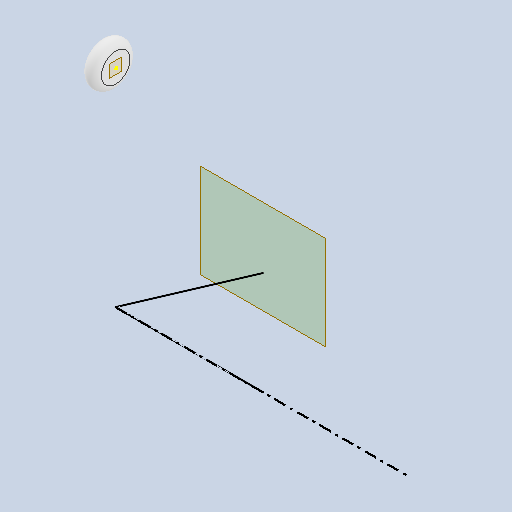
# Autodesk Inventor part: Landing Gear Wheel
Saved by Autodesk Inventor 2025 (Build 290162000, 162)
## iProperties
Created: 2024-09-17
Part Number: Landing Gear Wheel
Material: ABS Plastic
Document SubType Name: Modeling
Designer: Cupri
Density: 1.06 g/cm^3
Appearance: Smooth - White
Mass: 106.525 g
Surface Area: 124.48 cm^2
Volume: 100.495 cm^3
Author: Cupri
Autodesk Inventor part; units mm, degrees
ref_plane "YZ Plane" through (0, 0, 0) normal (1, 0, 0) x (0, 1, 0)
ref_plane "XZ Plane" through (0, 0, 0) normal (0, 1, 0) x (-1, 0, 0)
ref_plane "XY Plane" through (0, 0, 0) normal (0, 0, 1) x (1, 0, 0)
ref_plane "Work Plane1" through (199.3338, -160.5604, 1487.4212) normal (0, 0, -1) x (-1, 0, 0)
sketch "Sketch1" plane through (199.3338, -160.5604, 1487.4212) normal (0, 0, -1) x (-1, 0, 0)
  line L0 (-63.5, -25.4) -> (199.4935, -209.55) construction
  line L1 (199.4935, -209.55) -> (-326.4935, -209.55)
  line L2 (-63.5, -25.4) -> (199.4935, -209.55)
  line L3 (199.4935, -209.55) -> (-63.5, -209.55)
  point P0 (199.3338, 160.5604)
  constraints: 8 end point, 1 horizontal, 1 midpoint, 4 other
ref_plane "Work Plane2" through (0, 0, 1487.4212) normal (1, 0, 0) x (0, 1, 0)
sketch "Sketch4" plane through (0, 0, 1487.4212) normal (1, 0, 0) x (0, 1, 0)
  circle A0 centre (0, 0) radius 38.1
  point P0 (0, -1487.4212)
  dimension "d2" = 76.2
  constraints: 1 centre point
  measures "d2" diameter of A0
extrude "Extrusion1" add sketch "Sketch4" against normal blind 25.4
fillet "Fillet1" radius 12.7 2 edges at (-25.4, -38.1, 1487.4212) (0, -38.1, 1487.4212)
body "Solid1"
